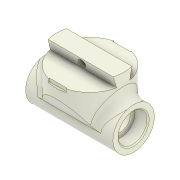
# Autodesk Inventor part: steering bottom half
Saved by Autodesk Inventor 2022 (Build 260153000, 153)
## iProperties
Created: 2024-03-23
Part Number: steering bottom half
Material: Generic
Document SubType Name: Modeling
Designer: david
Density: 1 g/cm^3
Appearance: Smooth - Ivory
Author: david
Autodesk Inventor part; units mm, degrees
ref_plane "YZ Plane" through (0, 0, 0) normal (1, 0, 0) x (0, 1, 0)
ref_plane "XZ Plane" through (0, 0, 0) normal (0, 1, 0) x (-1, 0, 0)
sketch "Sketch1" plane through (0, 0, 0) normal (0, 1, 0) x (-1, 0, 0)
  circle A0 centre (0, 0) radius 10.5 construction
  circle A1 centre (0, 0) radius 15.5
  dimension "hornDia" = 21
  dimension "d1" = 5
  constraints: 2 centre point, 1 coincident
  measures "hornDia" diameter of A0
  measures "d1" radial gap between concentric circles of A1 A0
extrude "Extrusion1" add sketch "Sketch1" against normal blind 24.25
sketch "Sketch2" plane through (0, 0, 0) normal (1, 0, 0) x (0, 1, 0)
  circle A0 centre (-24.25, 0) radius 6.5 construction
  line L0 (-35.1, 0) -> (5.85, 0) construction
  line L1 (-24.25, 15.5) -> (0, 15.5) construction
  line L2 (0, 15.5) -> (0, -15.5) construction
  line L3 (0, -15.5) -> (-24.25, -15.5) construction
  line L4 (-24.25, -15.5) -> (-24.25, 15.5) construction
  circle A1 centre (-24.25, 0) radius 9.5
  line L5 (-24.25, 15.5) -> (0, 15.5) projected
  line L6 (0, 15.5) -> (0, -15.5) projected
  line L7 (0, -15.5) -> (-24.25, -15.5) projected
  line L8 (-24.25, -15.5) -> (-24.25, 15.5) projected
  point P0 (0, 0)
  point P1 (0, 0)
  dimension "shaft" = 13
  dimension "d5" = 3
  constraints: 2 centre point, 2 midpoint, 1 horizontal alignment, 1 point on line
  measures "shaft" diameter of A0
  measures "d5" radial gap between concentric circles of A1 A0
extrude "Extrusion2" add sketch "Sketch2" along normal mid plane 40 contours A1 L8 | L8 A1
sketch "Sketch4" plane through (0, 0, 0) normal (0, 1, 0) x (1, 0, 0)
  circle A0 centre (0, 0) radius 12
  circle A1 centre (0, 0) radius 15.5 projected
  dimension "d15" = 24
  constraints: 1 centre point, 1 coincident
  measures "d15" diameter of A0
sketch "Sketch3" plane through (20, -24.25, 0) normal (1, 0, 0) x (0, 0, -1)
  circle A0 centre (0, 0) radius 9.5 projected
  point P0 (0, 24.25)
  constraints: 1 coincident
hole "Hole1" at (20, -24.25, 0) direction (-1, 0, 0) diameter 13 depth 6
mirror "Mirror1" about plane through (0, 0, 0) normal (1, 0, 0) of "Hole1"
sketch "Sketch9" plane through (14, -24.25, 0) normal (1, 0, 0) x (0, 0, -1)
  circle A0 centre (0, 0) radius 6.5 projected
  point P0 (0, 24.25)
  constraints: 1 coincident
hole "Hole5" at (14, -24.25, 0) direction (-1, 0, 0) diameter 9 end through all
thicken "Thicken1" operation add thickness 0.15 both sides no extend neighbours yes toward (0, 0.0804666, -0.9967573) faces at (18, -23.727, -6.4789)
extrude "Extrusion3" add sketch "Sketch4" along normal blind 5
sketch "Sketch5" plane through (0, 0, 0) normal (1, 0, 0) x (0, 1, 0)
  arc A0 (-24.25, 9.5) -> (-24.25, -9.5) centre (-24.25, 0) ccw projected
  line L0 (-24.25, 9.5) -> (-24.25, 15.5) projected
  line L1 (-24.25, 15.5) -> (5, 15.5) projected
  line L2 (5, 15.5) -> (5, 12) projected
  line L3 (5, 12) -> (0, 12) projected
  line L4 (0, 12) -> (0, -12) projected
  line L5 (0, -12) -> (5, -12) projected
  line L6 (5, -12) -> (5, -15.5) projected
  line L7 (5, -15.5) -> (-24.25, -15.5) projected
  line L8 (-24.25, -15.5) -> (-24.25, -9.5) projected
  circle A1 centre (-24.25, 0) radius 9.5 construction
  line L9 (5, 15.5) -> (-24.25, 15.5) projected
  line L10 (-14.75, 15.5) -> (-14.75, -15.5)
  line L11 (-24.25, 15.5) -> (-24.25, 9.5) projected
  line L12 (-14.75, 15.5) -> (-24.25, 9.5)
  line L13 (-24.25, -9.5) -> (-14.75, -15.5)
  circle A2 centre (-24.25, 0) radius 4.5 projected
  point P0 (0, 0)
  constraints: 6 end point, 2 point on line, 1 coincident, 1 perpendicular, 1 vertical, 1 vertical alignment, 2 other
extrude "Extrusion4" cut sketch "Sketch5" along normal through all both and the other way through all contours L0 L1 L12 | L13 L7 L8
fillet "Fillet1" radius 5 4 edges at (13.7186, -18.0695, -7.2146) (13.7186, -18.0694, 7.2146) (-13.7186, -18.0695, -7.2146) (-13.7184, -18.0698, 7.2149)
sketch "Sketch6" plane through (0, 0, 0) normal (0, 1, 0) x (1, 0, 0)
  circle A0 centre (0, 0) radius 7.5 construction
  line L0 (-28, 0) -> (28, 0) projected
  line L1 (0, 21.7) -> (0, -21.7) projected
  point P0 (0, 7.5)
  point P1 (-7.5, 0)
  point P2 (0, -7.5)
  point P3 (7.5, 0)
  dimension "d21" = 15
  dimension "d24" = 360
  constraints: 1 coincident, 1 point on line, 1 vertical alignment, 7 other
hole "Hole2" at (0, 0, -7.5) at (-7.5, 0, 0) at (0, 0, 7.5) at (7.5, 0, 0) direction (0, -1, 0) diameter 2 depth 5 tip angle 118
sketch "Sketch7" plane through (0, 0, 0) normal (0, 1, 0) x (1, 0, 0)
  circle A0 centre (0, 0) radius 12 projected
  constraints: 1 coincident
hole "Hole3" at (0, 0, 0) direction (0, -1, 0) diameter 10 depth 2
chamfer "Chamfer1" distance 2 angle 45 1 edges at (-12, 5, 0)
chamfer "Chamfer2" distance 0.5 angle 45 2 edges at (20, -24.25, 6.65) (-20, -24.25, 6.5)
ref_plane "Work Plane1" through (0, -9, 0) normal (0, 1, 0) x (1, 0, 0)
split body "Split1" result two bodies by plane through (0, -9, 0) normal (0, 1, 0) first body at (-14.9514, -6, -1.207)
sketch "Sketch21" plane through (0, -9, 0) normal (0, 1, 0) x (1, 0, 0)
  circle A0 centre (0, 0) radius 15.5 projected
  line L0 (14.8324, 4.5) -> (-14.8324, 4.5)
  line L1 (-14.8324, 4.5) -> (-14.8324, -4.5)
  line L2 (-14.8324, -4.5) -> (14.8324, -4.5)
  line L3 (14.8324, -4.5) -> (14.8324, 4.5)
  line L4 (14.8324, 4.5) -> (-14.8324, -4.5) construction
  line L5 (-14.8324, 4.5) -> (14.8324, -4.5) construction
  point P0 (4.5, 14.8324)
  point P1 (-14.8324, 4.5)
  point P2 (14.8324, -4.5)
  dimension "d110" = 9
  constraints: 12 end point, 2 midpoint, 2 parallel, 2 point on circle, 1 horizontal, 1 perpendicular
  measures "d110" distance of L0.end L1.end
extrude "Extrusion8" add sketch "Sketch21" along normal blind 5 contours A0 L3 | L3 L2 L1 L0 | L1 A0 bodies 3
sketch "Sketch23" plane through (0, 0, 0) normal (1, 0, 0) x (0, 1, 0)
  line L0 (-4, -4.5) -> (-4, 4.5) projected
  line L1 (-4, 4.5) -> (-9, 3.25)
  line L2 (-4, -4.5) -> (-9, -3.25)
  line L3 (-9, -4.5) -> (-4, -4.5) projected
  line L4 (-9, -4.5) -> (-9, 4.5)
  line L5 (-9, 15.5) -> (-9, 4.5) projected
  line L6 (-41.5, 0) -> (12.75, 0) projected
  line L7 (-9, 4.5) -> (-4, 4.5) projected
  point P0 (0, 0)
  dimension "d112" = 6.5
  constraints: 6 end point, 2 point on line, 1 other
  measures "d112" distance of L1.end L2.end
extrude "Extrusion10" cut sketch "Sketch23" along normal through all both and the other way through all contours L3 L4 L2 | L1 L4 L7 bodies 3
ref_plane "Work Plane5" through (0, 0, 15.5) normal (0, 0, 1) x (1, 0, 0)
sketch "Sketch24" plane through (0, 0, 15.5) normal (0, 0, 1) x (1, 0, 0)
  ellipse E0 centre (0, -22) end of major axis (0, -84) minor radius 15.5 (15.1554, -9) -> (14.8324, -4) ccw projected
  line L0 (-14.8324, -4) -> (14.8324, -4) projected
  ellipse E1 centre (0, -22) end of major axis (0, -84) minor radius 15.5 (-14.8324, -4) -> (-15.1554, -9) ccw projected
  line L1 (-15.1554, -9) -> (15.1554, -9) projected
  line L2 (15.5, -4) -> (14.8324, -4) projected
  line L3 (-14.8324, -4) -> (14.8324, -4) projected
  line L4 (0, -4) -> (0, -9)
  line L5 (-15.1554, -9) -> (15.1554, -9) projected
  point P0 (0, 0)
  point P1 (0, -6.5)
  constraints: 3 midpoint, 2 end point, 2 other
hole "Hole9" at (0, -6.5, 15.5) direction (0, 0, -1) diameter 3.4 end through all bodies 3
sketch "Sketch25" plane through (0, 0, 15.5) normal (0, 0, 1) x (1, 0, 0)
  line L0 (-15.1554, -9) -> (15.1554, -9) projected
  line L1 (-14.8324, -4) -> (14.8324, -4) projected
  line L2 (0, -4) -> (0, -9)
  line L3 (-15.1554, -9) -> (15.1554, -9) projected
  line L4 (-4, -10.5) -> (4, -10.5)
  line L5 (4, -10.5) -> (4, -2.5)
  line L6 (4, -2.5) -> (-4, -2.5)
  line L7 (-4, -2.5) -> (-4, -10.5)
  line L8 (-4, -10.5) -> (4, -2.5) construction
  line L9 (4, -10.5) -> (-4, -2.5) construction
  point P0 (0, 0)
  point P1 (0, -6.5)
  point P2 (4, -4)
  point P3 (-4, -4)
  dimension "d123" = 8
  dimension "d124" = 8
  constraints: 14 end point, 5 midpoint, 2 parallel, 1 horizontal, 1 perpendicular
  measures "d123" distance of L6.end L5.end
  measures "d124" distance of L5.end L4.end
extrude "Extrusion11" cut sketch "Sketch25" against normal blind 1 contours L7 L1 L2 L0 | L0 L5 L4 L7 | L2 L1 L5 L0 bodies 3
mirror "Mirror2" about plane through (0, 0, 15.5) normal (0, 0, 1) of "Extrusion11" bodies 3
sketch "Sketch26" plane through (0, 0, 0) normal (1, 0, 0) x (0, 1, 0)
  line L0 (-4, -4.5) -> (-4, 4.5) projected
  line L1 (-4, -4.5) -> (-9, -3.25) projected
  line L2 (-9, 3.25) -> (-4, 4.5) projected
  line L3 (-9, -3.25) -> (-9, -15.5) projected
  line L4 (-9, 3.25) -> (-9, -3.25)
  line L5 (-4.2, 4.2438) -> (-4.2, -4.2438)
  line L6 (-4.2, -4.2438) -> (-8.8, -3.0938)
  line L7 (-8.8, -3.0938) -> (-8.8, 3.0938)
  line L8 (-8.8, 3.0938) -> (-4.2, 4.2438)
  line L9 (-8.8, -3.0938) -> (-9, -3.0438)
  line L10 (-8.8, 3.0938) -> (-9, 3.0438)
  point P0 (0, 0)
  dimension "d127" = 0.2
  constraints: 14 end point, 3 collinear, 2 point on line, 3 other
  measures "d127" distance between parallel lines of L0 L5
extrude "Extrusion12" cut sketch "Sketch26" along normal through all both and the other way through all contours L1 L4 L9 L6 L5 L8 L10 L2 L0 bodies 3
mirror "Mirror3" about plane through (0, 0, 0) normal (0, 0, 1) of "Extrusion11" bodies 3
equation "\"d8\" = shaft"
equation "\"d124\" = d123"
body "Solid2"
body "Solid3"
